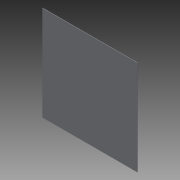
# Autodesk Inventor part: floor
Saved by Autodesk Inventor 2013 (Build 170138000, 138)
## iProperties
Created: 2011-06-21
Part Number: floor
Document SubType Name: Modeling
Designer: rrw
Density: 1 g/cm^3
Material: Generic
Author: rrw
Autodesk Inventor part; units mm, degrees
ref_plane "YZ Plane" through (0, 0, 0) normal (1, 0, 0) x (0, 1, 0)
ref_plane "XZ Plane" through (0, 0, 0) normal (0, 1, 0) x (-1, 0, 0)
ref_plane "XY Plane" through (0, 0, 0) normal (0, 0, 1) x (1, 0, 0)
sketch "Sketch1" plane through (0, 0, 0) normal (0, 0, 1) x (1, 0, 0)
  line L0 (-1143.2306, 1291.3637) -> (1656.7694, 1291.3637)
  line L1 (1656.7694, 1291.3637) -> (1656.7694, -1508.6363)
  line L2 (1656.7694, -1508.6363) -> (-1143.2306, -1508.6363)
  line L3 (-1143.2306, -1508.6363) -> (-1143.2306, 1291.3637)
  point P0 (0, 0)
  dimension "d0" = 2800
  dimension "d1" = 2800
  constraints: 8 end point, 2 parallel, 1 horizontal, 1 perpendicular
  measures "d0" distance of L1.end L2.end
  measures "d1" distance of L0.end L1.end
extrude "Extrusion1" add sketch "Sketch1" along normal blind 10
body "Solid1"
